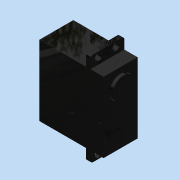
# Autodesk Inventor part: HitecServoBody
Saved by Autodesk Inventor 2017 (Build 210142000, 142)
## iProperties
Created: 2014-01-17
Part Number: HitecServoBody
Material: ABS Plastic
Document SubType Name: Modeling
Designer: Derek
Density: 1.06 g/cm^3
Appearance: Smooth - Black
Author: Derek
Autodesk Inventor part; units mm, degrees
ref_plane "YZ Plane" through (0, 0, 0) normal (1, 0, 0) x (0, 1, 0)
ref_plane "XZ Plane" through (0, 0, 0) normal (0, 1, 0) x (-1, 0, 0)
ref_plane "XY Plane" through (0, 0, 0) normal (0, 0, 1) x (1, 0, 0)
sketch "Sketch1" plane through (0, 0, 0) normal (0, 0, 1) x (1, 0, 0)
  line L0 (0, 0) -> (0, -40.64)
  line L1 (0, -40.64) -> (26.924, -40.64)
  line L2 (0, 0) -> (26.924, 0)
  line L3 (26.924, -40.64) -> (26.924, -47.244)
  line L4 (26.924, -47.244) -> (29.464, -47.244)
  line L5 (29.464, -47.244) -> (29.464, -40.64)
  line L6 (26.924, 0) -> (26.924, 6.604)
  line L7 (26.924, 6.604) -> (29.464, 6.604)
  line L8 (29.464, 6.604) -> (29.464, 0)
  line L9 (29.464, 0) -> (37.084, 0)
  line L10 (29.464, -40.64) -> (37.084, -40.64)
  line L11 (37.084, 0) -> (37.084, -40.64)
  dimension "d0" = 40.64
  dimension "d4" = 6.604
  dimension "d45" = 2.54
  dimension "d46" = 26.924
  dimension "d47" = 7.62
  dimension "d60" = 53.848
  constraints: 24 end point, 6 perpendicular, 5 equal length, 3 parallel, 2 horizontal, 1 coincident, 1 point on line, 1 vertical
  measures "d0" distance of L0.start L0.end
  measures "d4" distance of L2.end L6.end
  measures "d45" distance of L6.end L7.end
  measures "d46" distance of L0.start L2.end
  measures "d47" distance of L8.end L9.end
  measures "d60" distance between parallel lines of L4 L7
extrude "Extrusion8" add sketch "Sketch1" along normal blind 19.6342
sketch "Sketch8" plane through (37.084, -40.64, 0) normal (1, 0, 0) x (0, 0, -1)
  line L0 (0, 0) -> (0, 40.64) projected
  line L1 (0, 40.64) -> (-19.6342, 40.64) projected
  line L2 (-19.6342, 0) -> (-19.6342, 40.64) projected
  line L3 (0, 0) -> (-19.6342, 0) projected
  circle A0 centre (-9.8171, 30.861) radius 6.477
  dimension "d50" = 12.954
  dimension "d51" = 9.779
  constraints: 1 centre point
  measures "d50" diameter of A0
  measures "d51" distance from line of L1 A0.centre
extrude "Extrusion9" add sketch "Sketch8" along normal blind 1.778 contours A0
sketch "Sketch9" plane through (29.464, 0, 0) normal (1, 0, 0) x (0, 0, -1)
  circle A0 centre (-14.8971, 3.81) radius 2.1082
  line L0 (0, 6.604) -> (-19.6342, 6.604) projected
  line L1 (-9.8171, 6.604) -> (-9.8171, 8.0872)
  line L2 (0, 0) -> (-19.6342, 0) projected
  circle A1 centre (-4.7371, 3.81) radius 2.1082
  line L3 (0, 0) -> (0, -40.64) projected
  line L4 (0, -20.32) -> (8.7495, -20.32)
  circle A2 centre (-14.8971, -44.45) radius 2.1082
  circle A3 centre (-4.7371, -44.45) radius 2.1082
  dimension "d54" = 4.2164
  dimension "d55" = 5.08
  dimension "d56" = 3.81
  constraints: 4 centre point, 4 end point, 3 symmetric about line, 2 midpoint, 1 horizontal, 1 vertical, 3 other
  measures "d54" diameter of A0
  measures "d55" distance from line of L1 A0.centre
  measures "d56" distance from line of A0.centre L2
extrude "Extrusion10" cut sketch "Sketch9" against normal through all
fillet "Fillet1" radius 1.524 4 edges at (28.194, 6.604, 19.6342) (28.194, 6.604, 0) (28.194, -47.244, 19.6342) (28.194, -47.244, 0)
body "Solid2"
